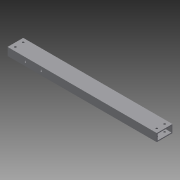
# Autodesk Inventor part: 2x1 support horizontal
Saved by Autodesk Inventor 2015 SP1 (Build 190203100, 203)
## iProperties
Created: 2015-01-16
Part Number: 2x1 support horizontal
Material: Generic
Document SubType Name: Modeling
Designer: 215152
Density: 1 g/cm^3
Appearance: Default
Author: 215152
Autodesk Inventor part; units mm, degrees
ref_plane "YZ Plane" through (0, 0, 0) normal (1, 0, 0) x (0, 1, 0)
ref_plane "XZ Plane" through (0, 0, 0) normal (0, 1, 0) x (-1, 0, 0)
ref_plane "XY Plane" through (0, 0, 0) normal (0, 0, 1) x (1, 0, 0)
sketch "Sketch1" plane through (0, 0, 0) normal (1, 0, 0) x (0, 1, 0)
  line L0 (0, 0) -> (25.4, 0)
  line L1 (25.4, 0) -> (25.4, -50.8)
  line L2 (25.4, -50.8) -> (0, -50.8)
  line L3 (0, -50.8) -> (0, 0)
  line L4 (3.175, -3.175) -> (22.225, -3.175)
  line L5 (22.225, -3.175) -> (22.225, -47.625)
  line L6 (22.225, -47.625) -> (3.175, -47.625)
  line L7 (3.175, -47.625) -> (3.175, -3.175)
  dimension "d0" = 25.4
  dimension "d1" = 50.8
  dimension "d2" = 19.05
  dimension "d3" = 44.45
  dimension "d4" = 3.175
  dimension "d5" = 3.175
  constraints: 16 end point, 4 parallel, 2 horizontal, 2 perpendicular
  measures "d0" distance of L1.end L2.end
  measures "d1" distance of L0.end L1.end
  measures "d2" distance of L5.end L6.end
  measures "d3" distance of L4.end L5.end
  measures "d4" distance between parallel lines of L3 L7
  measures "d5" distance between parallel lines of L0 L4
extrude "Extrusion1" add sketch "Sketch1" along normal blind 482.6
sketch "Sketch2" plane through (0, 25.4, 0) normal (0, 1, 0) x (1, 0, 0)
  line L0 (0, 0) -> (0, 50.8) projected
  line L1 (0, 0) -> (482.6, 0) projected
  line L2 (482.6, 50.8) -> (482.6, 0) projected
  line L3 (0, 50.8) -> (482.6, 50.8) projected
  point P0 (12.7, 12.7)
  point P1 (12.7, 38.1)
  point P2 (469.9, 12.7)
  point P3 (469.9, 38.1)
  dimension "d8" = 12.7
  dimension "d9" = 12.7
  dimension "d10" = 12.7
  dimension "d11" = 12.7
  dimension "d12" = 12.7
  dimension "d13" = 12.7
  dimension "d14" = 12.7
  dimension "d15" = 12.7
  measures "d8" distance from line of L2 point (469.9, 12.7)
  measures "d9" distance from line of L1 point (469.9, 12.7)
  measures "d10" distance from line of L3 point (469.9, 38.1)
  measures "d11" distance from line of L2 point (469.9, 38.1)
  measures "d12" distance from line of L0 point (12.7, 38.1)
  measures "d13" distance from line of L3 point (12.7, 38.1)
  measures "d14" distance from line of L1 point (12.7, 12.7)
  measures "d15" distance from line of L0 point (12.7, 12.7)
hole "Hole1" at (12.7, 25.4, -12.7) at (12.7, 25.4, -38.1) at (469.9, 25.4, -12.7) at (469.9, 25.4, -38.1) direction (0, -1, 0) diameter 6.35 end through all
sketch "Sketch3" plane through (0, 0, 0) normal (0, 0, 1) x (1, 0, 0)
  line L0 (0, 0) -> (0, 25.4) projected
  line L1 (0, 0) -> (482.6, 0) projected
  line L2 (482.6, 25.4) -> (482.6, 0) projected
  line L3 (0, 25.4) -> (482.6, 25.4) projected
  point P0 (57.15, 12.7)
  point P1 (107.95, 12.7)
  dimension "d23" = 57.15
  dimension "d24" = 12.7
  dimension "d25" = 12.7
  dimension "d26" = 107.95
  measures "d23" distance from line of L0 point (57.15, 12.7)
  measures "d24" distance from line of L1 point (57.15, 12.7)
  measures "d25" distance from line of L1 point (107.95, 12.7)
  measures "d26" distance from line of L0 point (107.95, 12.7)
hole "Hole2" at (57.15, 12.7, 0) at (107.95, 12.7, 0) direction (0, 0, -1) diameter 6.35 end through all
body "Solid1"
